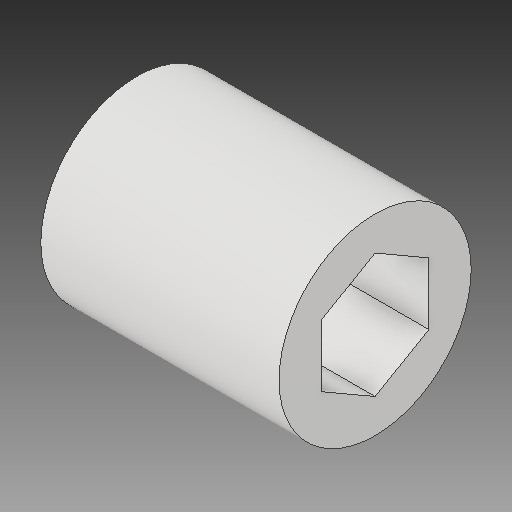
# Autodesk Inventor part: Mec Wheel Spacer
Saved by Autodesk Inventor 2019.4 (Build 234330000, 330)
## iProperties
Created: 2020-01-29
Part Number: Mec Wheel Spacer
Material: ABS Plastic
Document SubType Name: Modeling
Designer: admin
Density: 1.06 g/cm^3
Appearance: Smooth - White
Mass: 2.27932 g
Surface Area: 16.4895 cm^2
Volume: 2.15031 cm^3
Author: admin
Autodesk Inventor part; units mm, degrees
ref_plane "YZ Plane" through (0, 0, 0) normal (1, 0, 0) x (0, 1, 0)
ref_plane "XZ Plane" through (0, 0, 0) normal (0, 1, 0) x (-1, 0, 0)
ref_plane "XY Plane" through (0, 0, 0) normal (0, 0, 1) x (1, 0, 0)
sketch "Sketch1" plane through (0, 0, 0) normal (1, 0, 0) x (0, 1, 0)
  line L0 (-2.4249, 4.2) -> (2.4249, 4.2)
  line L1 (2.4249, 4.2) -> (4.8497, 0)
  line L2 (4.8497, 0) -> (2.4249, -4.2)
  line L3 (2.4249, -4.2) -> (-2.4249, -4.2)
  line L4 (-2.4249, -4.2) -> (-4.8497, 0)
  line L5 (-4.8497, 0) -> (-2.4249, 4.2)
  circle A0 centre (0, 0) radius 7.5
  dimension "d0" = 8.4
  dimension "d1" = 15
  constraints: 12 end point, 2 coincident, 1 centre point, 1 horizontal, 13 other
  measures "d0" distance between parallel lines of L3 L0
  measures "d1" diameter of A0
extrude "Extrusion1" add sketch "Sketch1" along normal blind 18.6
body "Solid1"
